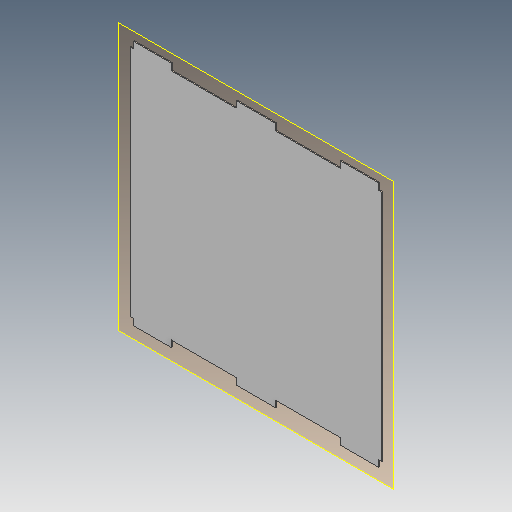
# Autodesk Inventor part: lr_heater
Saved by Autodesk Inventor 2020 (Build 240168000, 168)
## iProperties
Created: 2021-05-08
Part Number: lr_heater
Material: Generic
Document SubType Name: Modeling
Designer: Hsu Daniel
Density: 1 g/cm^3
Appearance: Default
Author: Hsu Daniel
Autodesk Inventor part; units mm, degrees
ref_plane "YZ Plane" through (0, 0, 0) normal (1, 0, 0) x (0, 1, 0)
ref_plane "XZ Plane" through (0, 0, 0) normal (0, 1, 0) x (-1, 0, 0)
sketch "Sketch1" plane through (0, 0, 0) normal (0, 0, 1) x (1, 0, 0)
  line L0 (0, 0) -> (126.6, 0)
  line L1 (1.7, 0) -> (1.7, -3.3)
  line L2 (1.7, -3.3) -> (20.7, -3.3)
  line L3 (20.7, -3.3) -> (20.7, 0)
  line L4 (53.35, 0) -> (53.35, -3.3)
  line L5 (53.35, -3.3) -> (73.25, -3.3)
  line L6 (73.25, -3.3) -> (73.25, 0)
  line L7 (105.9, 0) -> (105.9, -3.3)
  line L8 (105.9, -3.3) -> (124.9, -3.3)
  line L9 (124.9, -3.3) -> (124.9, 0)
  line L10 (11.2, -3.3) -> (11.2, 0) construction
  line L11 (63.3, -3.3) -> (63.3, 0) construction
  line L12 (115.4, -3.3) -> (115.4, 0) construction
  line L13 (63.3, 0) -> (63.3, 12.1181) construction
  line L14 (0, 0) -> (0, 58.65)
  line L15 (0, 58.65) -> (126.6, 58.65) construction
  line L16 (126.6, 0) -> (126.6, 58.65)
  line L17 (0, 117.3) -> (126.6, 117.3)
  line L18 (1.7, 117.3) -> (1.7, 120.6)
  line L19 (1.7, 120.6) -> (20.7, 120.6)
  line L20 (20.7, 120.6) -> (20.7, 117.3)
  line L21 (53.35, 117.3) -> (53.35, 120.6)
  line L22 (53.35, 120.6) -> (73.25, 120.6)
  line L23 (73.25, 120.6) -> (73.25, 117.3)
  line L24 (105.9, 117.3) -> (105.9, 120.6)
  line L25 (105.9, 120.6) -> (124.9, 120.6)
  line L26 (124.9, 120.6) -> (124.9, 117.3)
  line L27 (11.2, 120.6) -> (11.2, 117.3) construction
  line L28 (63.3, 120.6) -> (63.3, 117.3) construction
  line L29 (115.4, 120.6) -> (115.4, 117.3) construction
  line L30 (63.3, 117.3) -> (63.3, 105.1819) construction
  line L31 (0, 117.3) -> (0, 58.65)
  line L32 (126.6, 117.3) -> (126.6, 58.65)
  dimension "d12" = 126.6
  dimension "d13" = 3.3
  dimension "d14" = 19
  dimension "d15" = 3.3
  dimension "d16" = 19.9
  dimension "d17" = 3.3
  dimension "d18" = 19
  dimension "d19" = 52.1
  dimension "d20" = 52.1
  dimension "d21" = 58.65
  constraints: 62 end point, 22 symmetric about line, 11 vertical, 4 point on line, 3 midpoint, 3 perpendicular, 1 collinear, 25 other
  measures "d12" distance of L14.start L16.start
  measures "d13" distance of L1.start L1.end
  measures "d14" distance of L1.end L2.end
  measures "d15" distance of L4.start L4.end
  measures "d16" distance of L4.end L5.end
  measures "d17" distance of L7.start L7.end
  measures "d18" distance of L7.end L8.end
  measures "d19" distance between parallel lines of L11 L10
  measures "d20" distance between parallel lines of L12 L11
  measures "d21" distance of L14.start L14.end
extrude "Extrusion1" add sketch "Sketch1" along normal blind 0.5
ref_plane "Work Plane1" through (0, 0, 0.25) normal (0, 0, 1) x (1, 0, 0)
ref_plane "Work Plane2" through (63.3, 0, 0) normal (1, 0, 0) x (0, 0, -1)
equation "\"d12\" = lrltotal"
equation "\"d13\" = lrdepth"
equation "\"d14\" = lrlr"
equation "\"d15\" = lrdepth"
equation "\"d16\" = lrmid"
equation "\"d17\" = lrdepth"
equation "\"d18\" = lrlr"
equation "\"d20\" = d19"
equation "\"d21\" = 0.5 * heaterH"
equation "\"d22\" = thick"
equation "\"thick\" = 0.5"
equation "\"lrlr\" = 19"
equation "\"lrmid\" = 19.9"
equation "\"lrdepth\" = 3.3"
equation "\"mlr\" = 16.6"
equation "\"mmid\" = 24.7"
equation "\"mdepth\" = 4.5"
equation "\"lrltotal\" = 126.6"
equation "\"mltotal\" = 126.6"
equation "\"lrbetween\" = 52.1"
equation "\"mbetween\" = 49.5"
equation "\"toler\" = 1"
equation "\"stuckw\" = 6"
equation "\"tight\" = 0.08"
equation "\"sidewallL\" = 132.6"
equation "\"heaterH\" = 117.3"
equation "\"stickL\" = 3.5"
equation "\"wireH\" = 25"
body "Solid1"
